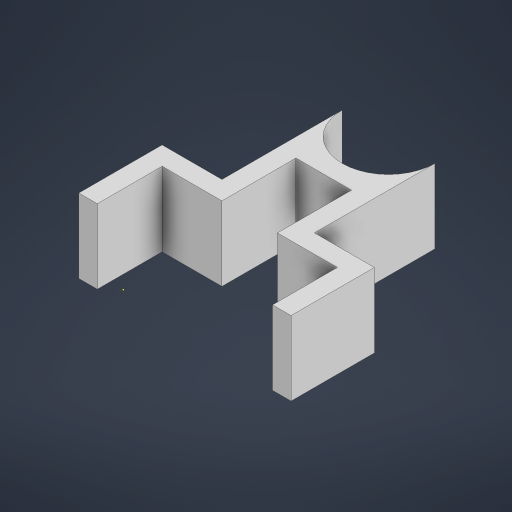
# Autodesk Inventor part: Część4
Saved by Autodesk Inventor 2023 (Build 270158000, 158)
## iProperties
Created: 2023-05-07
Part Number: Część4
Material: Ogólny
Document SubType Name: Modeling
Designer: Adam
Density: 1 g/cm^3
Appearance: Domyślna
Author: Adam
Autodesk Inventor part; units mm, degrees
ref_plane "YZ Plane" through (0, 0, 0) normal (1, 0, 0) x (0, 1, 0)
ref_plane "XZ Plane" through (0, 0, 0) normal (0, 1, 0) x (-1, 0, 0)
ref_plane "XY Plane" through (0, 0, 0) normal (0, 0, 1) x (1, 0, 0)
sketch "Szkic1" plane through (0, 0, 0) normal (0, 1, 0) x (-1, 0, 0)
  circle A0 centre (0, -143.2209) radius 25
  line L0 (25, -143.2209) -> (25, -78.2209)
  line L1 (25, -78.2209) -> (57.3466, -78.2209)
  line L2 (57.3466, -78.2209) -> (57.3466, -33.2209)
  line L3 (57.3466, -33.2209) -> (47.3466, -33.2209)
  line L4 (47.3466, -33.2209) -> (47.3466, -68.2209)
  line L5 (47.3466, -68.2209) -> (15, -68.2209)
  line L6 (15, -68.2209) -> (15, -108.2209)
  line L7 (15, -108.2209) -> (0, -108.2209)
  line L8 (0, -108.2209) -> (0, 0)
  line L9 (-25, -143.2209) -> (-25, -78.2209)
  line L10 (-25, -78.2209) -> (-57.3466, -78.2209)
  line L11 (-57.3466, -78.2209) -> (-57.3466, -33.2209)
  line L12 (-57.3466, -33.2209) -> (-47.3466, -33.2209)
  line L13 (-47.3466, -33.2209) -> (-47.3466, -68.2209)
  line L14 (-47.3466, -68.2209) -> (-15, -68.2209)
  line L15 (-15, -68.2209) -> (-15, -108.2209)
  line L16 (-15, -108.2209) -> (0, -108.2209)
  point P0 (7.5, -108.2209)
  point P1 (52.3466, -33.2209)
  dimension "d0" = 50
  dimension "d1" = 35
  dimension "d2" = 65
  dimension "d3" = 10
  dimension "d4" = 45
  dimension "d5" = 15
  dimension "d6" = 10
  dimension "d7" = 10
  constraints: 34 end point, 8 symmetric about line, 6 perpendicular, 3 vertical, 2 midpoint, 1 horizontal, 3 other
  measures "d1" vertical distance of point (7.5, -108.221) point (0, -143.221)
  measures "d2" distance from line of point (0, -143.221) L1
  measures "d3" distance between parallel lines of L5 L1
  measures "d4" distance from line of point (52.347, -33.221) L1
  measures "d5" distance of L6.end L7.end
  measures "d6" distance between parallel lines of L6 L0
  measures "d7" distance between parallel lines of L4 L2
extrude "Wyciągnięcie proste1" add sketch "Szkic1" along normal blind 40 contours A0 L9 L10 L11 L12 L13 L14 L15 L16 L7 L6 L5 L4 L3 L2 L1 L0
sketch "Szkic2" plane through (0, 40, 0) normal (0, 1, 0) x (1, 0, 0)
  point P0 (0, 0)
